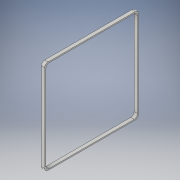
# Autodesk Inventor part: Coil3or4
Saved by Autodesk Inventor 2019 (Build 230136000, 136)
## iProperties
Created: 2021-05-17
Part Number: Coil3or4
Material: Generic
Document SubType Name: Modeling
Designer: jamieson-bl
Density: 1 g/cm^3
Appearance: Default
Author: jamieson-bl
Autodesk Inventor part; units mm, degrees
ref_plane "YZ Plane" through (0, 0, 0) normal (1, 0, 0) x (0, 1, 0)
ref_plane "XZ Plane" through (0, 0, 0) normal (0, 1, 0) x (-1, 0, 0)
ref_plane "XY Plane" through (0, 0, 0) normal (0, 0, 1) x (1, 0, 0)
sketch "Sketch1" plane through (0, 0, 0) normal (1, 0, 0) x (0, 1, 0)
  line L0 (-910, -980) -> (910, -980)
  line L1 (980, -910) -> (980, 910)
  line L2 (910, 980) -> (-910, 980)
  line L3 (-980, 910) -> (-980, -910)
  line L4 (-980, -980) -> (980, 980) construction
  line L5 (980, -980) -> (-980, 980) construction
  line L6 (-885, -955) -> (885, -955)
  line L7 (955, -885) -> (955, 885)
  line L8 (885, 955) -> (-885, 955)
  line L9 (-955, 885) -> (-955, -885)
  line L10 (-955, -955) -> (955, 955) construction
  line L11 (955, -955) -> (-955, 955) construction
  arc A0 (885, -955) -> (955, -885) centre (885, -885) ccw
  arc A1 (910, -980) -> (980, -910) centre (910, -910) ccw
  arc A2 (-955, -885) -> (-885, -955) centre (-885, -885) ccw
  arc A3 (-980, -910) -> (-910, -980) centre (-910, -910) ccw
  arc A4 (-885, 955) -> (-955, 885) centre (-885, 885) ccw
  arc A5 (-910, 980) -> (-980, 910) centre (-910, 910) ccw
  arc A6 (955, 885) -> (885, 955) centre (885, 885) ccw
  arc A7 (980, 910) -> (910, 980) centre (910, 910) ccw
  point P0 (0, 0)
  dimension "d0" = 1960
  dimension "d1" = 1960
  dimension "d2" = 1910
  dimension "d3" = 1910
  dimension "d4" = 70
  constraints: 24 end point, 16 point on circle, 16 point on line, 16 tangent, 8 centre point, 7 equal radius, 4 midpoint, 4 parallel, 2 horizontal, 2 perpendicular
  measures "d0" distance of L5.end L4.end
  measures "d1" distance of L4.end L5.start
  measures "d2" distance of L11.end L10.end
  measures "d3" distance of L10.end L11.start
  measures "d4" radius of A0
extrude "Extrusion1" add sketch "Sketch1" along normal blind 70
body "Solid1"
